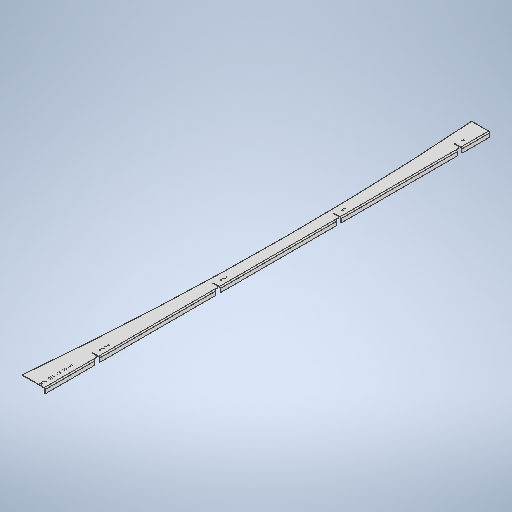
# Autodesk Inventor part: MSC 052 rib board
Saved by Autodesk Inventor 2025 (Build 290162010, 162A)
## iProperties
Created: 2024-04-28
Part Number: MSC 052 rib board
Material: Stainless Steel
Document SubType Name: Sheet Metal
Designer: admin
Density: 8 g/cm^3
Sheet Metal Rule: AISI304 2mm Die16
Appearance: Default
Flat Pattern Width: 184 cm
Flat Pattern Length: 11.2202 cm
Flat Pattern Area: 2064.52 cm^2
Sheet Metal Width: 1840,000 mm
Sheet Metal Length: 112,202 mm
Sheet Metal Area: 206451,663 mm^2
Stock Number: МОО 052 шпангоут борт
Description: DIE16(5)|\ 90°|corrY -15°|corrX -1.45|bom0,25
БОРТ_стрингер_3_высота: 67,000 mm
БОРТ_стрингер_4_высота: 48,000 mm
БОРТ_стрингер_5_высота: 51,000 mm
БОРТ_стрингер_6_высота: 77,000 mm
РЕБРА_глубина_паза: 30,000 mm
РЕБРА_вырез_на_полке: 5,000 mm
РЕБРА_полка: 20,000 mm
Author: admin
Autodesk Inventor part; units mm, degrees
ref_plane "YZ Plane" through (0, 0, 0) normal (1, 0, 0) x (0, 1, 0)
ref_plane "XZ Plane" through (0, 0, 0) normal (0, 1, 0) x (-1, 0, 0)
ref_plane "XY Plane" through (0, 0, 0) normal (0, 0, 1) x (1, 0, 0)
sketch "Sketch1" plane through (0, 0, 0) normal (0, 0, 1) x (1, 0, 0)
  arc A0 (-96, -1840) -> (-75, 0) centre (-11096.4126, -794.332) ccw
  line L0 (0, 0) -> (-75, 0)
  line L1 (0, -188.6809) -> (-63.023, -188.6809) construction
  line L2 (0, -688.6809) -> (-46.9177, -688.6809) construction
  line L3 (0, -1188.6809) -> (-53.4516, -1188.6809) construction
  line L4 (0, -1688.6809) -> (-82.6649, -1688.6809) construction
  line L5 (-96, -1840) -> (0, -1840)
  line L6 (0, 0) -> (0, -1840)
  point P0 (-25, 0)
  dimension "d33" = 50
  dimension "d58" = 500
  dimension "d59" = 500
  dimension "d60" = 500
  dimension "d141" = 1840
  dimension "d148" = 75
  dimension "d149" = 11050
  dimension "d150" = 96
  measures "d33" distance of L0.end point (-25, 0)
  measures "d58" distance between parallel lines of L2 L1
  measures "d59" distance between parallel lines of L2 L3
  measures "d60" distance between parallel lines of L3 L4
  measures "d141" distance between parallel lines of L0 L5
  measures "d148" distance of L0.start L0.end
  measures "d149" radius of A0
  measures "d150" distance of L5.start L5.end
extrude "Plate3" add sketch "Sketch1" along normal blind 2
sketch "Sketch3" plane through (-2, 0, 2) normal (1, 0, 0) x (0, 1, 0)
  line L0 (-1840, 0) -> (0, 0)
  line L1 (0, 0) -> (0, 20)
  line L2 (0, 20) -> (-1840, 20)
  line L3 (-1840, 20) -> (-1840, 0)
  constraints: 6 end point, 1 horizontal, 1 perpendicular, 1 vertical
edge flange "Flange2" height 20 angle 90 thickness 2 bend radius 2.75 thickness toward (1, 0, 0) relief round relief width 2 relief depth 1 edges at (0, -920, 2) wall of the first edge with corners at (-2, -1840, 2) (-2, 0, 2) (-2, 0, -18) (-2, -1840, -18)
bend "Bend2"
corner "Corner2"
sketch "Sketch5" plane through (0, 0, 0) normal (0, 0, 1) x (1, 0, 0)
  line L0 (-4.75, -1840) -> (-4.75, 0) projected
  line L1 (-75, 0) -> (-4.75, 0) projected
  arc A0 (-96, -1840) -> (-75, 0) centre (-11096.4126, -794.332) ccw projected
  line L2 (0, 0) -> (0, -1840) projected
  line L3 (0, -115) -> (-31, -115)
  line L4 (0, -117) -> (-2, -117) construction
  line L5 (-2, -1840) -> (-2, 0) projected
  line L6 (-31, -115) -> (-31, -117)
  line L7 (0, -615) -> (-47.8679, -615) construction
  line L8 (0, -1115) -> (-51.0665, -1115) construction
  line L9 (0, -1615) -> (-76.9297, -1615) construction
  line L10 (-4.75, -1840) -> (-96, -1840) projected
  line L11 (0, -115) -> (0, -135)
  line L12 (-2, -115) -> (-2, -117) construction
  line L13 (0, -135) -> (-2, -135)
  line L14 (-31, -115) -> (-67.3144, -115) construction
  line L15 (-31, -117) -> (-67.1914, -117) construction
  line L16 (-2, -117) -> (-2, -135)
  line L17 (-2, -117) -> (-31, -117)
  line L18 (-2, -135) -> (-4.75, -135)
  point P0 (845.25, -380.4205)
  point P1 (848, -380.4205)
  point P2 (-31, -116)
  point P3 (-2, -135)
  point P4 (850, -410.4205)
  point P5 (-2, -115)
  point P6 (-2, -135)
  point P7 (-4.75, -117)
  dimension "d69" = 1840
  dimension "d70" = 2
  dimension "d76" = 67.3144
  dimension "d80" = 47.8679
  dimension "d102" = 76.9297
  dimension "d104" = 51.0665
  dimension "d106" = 2
  dimension "d107" = 20
  dimension "d108" = 116
  dimension "d112" = 31
  dimension "d142" = 500
  dimension "d143" = 500
  dimension "d144" = 500
  constraints: 28 end point, 13 perpendicular, 10 point on line, 5 point on circle, 2 parallel, 1 horizontal, 1 midpoint
  measures "d69" distance of L2.start L2.end
  measures "d70" distance between parallel lines of L4 L3
  measures "d76" distance of L3.start L14.end
  measures "d80" distance of L7.start L7.end
  measures "d102" distance of L9.start L9.end
  measures "d104" distance of L8.end L8.start
  measures "d106" distance of L13.end L11.end
  measures "d107" distance of L11.end L3.start
  measures "d108" vertical distance of L2.start point (-31, -116)
  measures "d112" distance of L3.end L3.start
  measures "d142" distance between parallel lines of L7 L14
  measures "d143" distance between parallel lines of L7 L8
  measures "d144" distance between parallel lines of L9 L8
extrude "Extrusion2" cut sketch "Sketch5" along normal through all both and the other way through all contours L0 L17 L5 L18 | L17 L6 L3 L0 | L0 L3 L5 L17 | L5 L3 L2 L13
pattern_linear "Rectangular Pattern3" count 4 spacing 500 along (0, -1, 0) of "Extrusion2"
sketch "Sketch6" plane through (0, 0, 0) normal (0, 0, -1) x (-1, 0, 0)
  line L0 (33.166, -1835) -> (21.166, -1835) construction
  line L1 (21.166, -1835) -> (21.166, -1635) construction
  line L2 (21.166, -1635) -> (33.166, -1635) construction
  line L3 (33.166, -1635) -> (33.166, -1835) construction
  line L4 (96, -1840) -> (96, -1840) projected
  line L5 (33.166, -1540) -> (33.166, -1590) construction
  line L6 (33.166, -1590) -> (21.166, -1590) construction
  line L7 (21.166, -1590) -> (21.166, -1540) construction
  line L8 (21.166, -1540) -> (33.166, -1540) construction
  line L9 (4.75, -1615) -> (31, -1615) projected
  line L10 (33.166, -1040) -> (33.166, -1090) construction
  line L11 (33.166, -1090) -> (21.166, -1090) construction
  line L12 (21.166, -1090) -> (21.166, -1040) construction
  line L13 (21.166, -1040) -> (33.166, -1040) construction
  line L14 (33.166, -540) -> (33.166, -590) construction
  line L15 (33.166, -590) -> (21.166, -590) construction
  line L16 (21.166, -590) -> (21.166, -540) construction
  line L17 (21.166, -540) -> (33.166, -540) construction
  line L18 (33.166, -40) -> (33.166, -90) construction
  line L19 (33.166, -90) -> (21.166, -90) construction
  line L20 (21.166, -90) -> (21.166, -40) construction
  line L21 (21.166, -40) -> (33.166, -40) construction
  line L22 (4.75, -1115) -> (31, -1115) projected
  line L23 (4.75, -615) -> (31, -615) projected
  line L24 (4.75, -115) -> (31, -115) projected
  point P0 (0, 0)
  point P1 (4.75, -1840)
  dimension "d120" = 200
  dimension "d121" = 12
  dimension "d123" = 5
  dimension "d126" = 50
  dimension "d127" = 25
  dimension "d135" = 25
  dimension "d136" = 25
  dimension "d137" = 25
  constraints: 7 equal length, 4 collinear, 1 horizontal alignment, 10 other
  measures "d120" distance of L0.end L1.end
  measures "d121" distance of L1.end L2.end
  measures "d126" distance of L6.end L7.end
  measures "d127" distance between parallel lines of L9 L6
  measures "d135" distance between parallel lines of L22 L11
  measures "d136" distance between parallel lines of L23 L15
  measures "d137" distance between parallel lines of L24 L19
mark "Mark1"
chamfer "Corner Chamfer1" distance 6 angle 45 4 edges at (-4.75, -1617, 1) (-4.75, -1117, 1) (-4.75, -617, 1) (-4.75, -117, 1)
equation "\"d33\" = d25"
equation "\"БОРТ_стрингер_3_высота\" = 67"
equation "\"БОРТ_стрингер_4_высота\" = 48"
equation "\"БОРТ_стрингер_5_высота\" = 51"
equation "\"БОРТ_стрингер_6_высота\" = 77"
equation "\"d25\" = 50"
body "Solid2"
